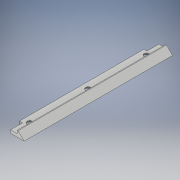
# Autodesk Inventor part: Plug
Saved by Autodesk Inventor 2019 (Build 230136000, 136)
## iProperties
Created: 2021-12-21
Part Number: Plug
Material: Ogólny
Document SubType Name: Modeling
Designer: Michał
Density: 1 g/cm^3
Appearance: Domyślna
Author: Michał
Autodesk Inventor part; units mm, degrees
ref_plane "YZ Plane" through (0, 0, 0) normal (1, 0, 0) x (0, 1, 0)
ref_plane "XZ Plane" through (0, 0, 0) normal (0, 1, 0) x (-1, 0, 0)
ref_plane "XY Plane" through (0, 0, 0) normal (0, 0, 1) x (1, 0, 0)
sketch "Szkic1" plane through (0, 0, 0) normal (0, 0, 1) x (1, 0, 0)
  line L0 (0, 0) -> (11, 0)
  line L1 (11, 0) -> (7, 4)
  line L2 (7, 4) -> (6.5, 4)
  line L3 (6.5, 4) -> (6.5, 2)
  line L4 (6.5, 2) -> (0, 2)
  line L5 (0, 2) -> (0, 0)
  dimension "d1" = 45
  dimension "d3" = 2
  dimension "d4" = 2
  dimension "d5" = 11
  dimension "d19" = 4.5
  constraints: 12 end point, 3 perpendicular, 1 horizontal, 1 parallel
  measures "d1" angle of L1 L0
  measures "d3" distance of L2.end L3.end
  measures "d4" distance of L4.end L0.start
  measures "d5" distance of L0.start L0.end
  measures "d19" distance from line of L0.end L3
extrude "Wyciągnięcie proste1" add sketch "Szkic1" against normal blind 98
sketch "Szkic4" plane through (0, 0, 0) normal (0, -1, 0) x (1, 0, 0)
  line L0 (0, 0) -> (0, -98) construction
  line L1 (0, -49) -> (11, -49) construction
  line L2 (11, 0) -> (11, -98) construction
  line L3 (4.3, -10.4) -> (4.3, -49) construction
  line L4 (6.5, 0) -> (6.5, -98) construction
  point P0 (4.3, -87.6)
  dimension "d10" = 2.2
  dimension "d11" = 38.6
  constraints: 4 end point, 2 midpoint, 1 perpendicular, 1 point on line, 1 symmetric about line
  measures "d10" distance between parallel lines of L4 L3
  measures "d11" distance of L3.start L3.end
hole "Otwór1" at (4.3, 0, -10.4) at (4.3, 0, -49) at (4.3, 0, -87.6) direction (0, 1, 0) diameter 3.4 end through all countersink diameter 6.9 countersink angle 84.225
sketch "Szkic5" plane through (0, 2, 0) normal (0, 1, 0) x (1, 0, 0)
  line L0 (0, 0) -> (11, 0) projected
  line L1 (0, 0) -> (2, 0)
  line L2 (2, 0) -> (2, 7.9)
  line L3 (2, 7.9) -> (0, 7.9)
  line L4 (0, 7.9) -> (0, 0)
  line L5 (0, 0) -> (0, 98) construction
  line L6 (0, 49) -> (11, 49) construction
  line L7 (11, 0) -> (11, 98) construction
  line L8 (6.5, 0) -> (6.5, 98) construction
  line L9 (0, 98) -> (2, 98)
  line L10 (2, 98) -> (2, 90.1)
  line L11 (2, 90.1) -> (0, 90.1)
  line L12 (0, 90.1) -> (0, 98)
  dimension "d20" = 4.5
  dimension "d21" = 7.9
  constraints: 18 end point, 3 symmetric about line, 2 midpoint, 2 parallel, 1 horizontal, 1 perpendicular
  measures "d20" distance between parallel lines of L2 L8
  measures "d21" distance of L3.end L0.start
extrude "Wyciągnięcie proste2" cut sketch "Szkic5" against normal through all
